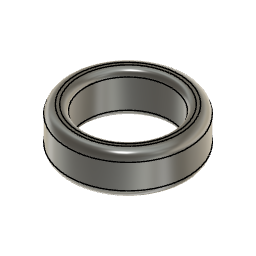
Anel_Redutor_Bracos_Imprimir (Autodesk Fusion 360 design; units mm, degrees)
Autodesk Fusion 360 part; units mm, degrees
sketch "Esboço1" plane through (0, 0, 0) normal (0, 0, 1) x (1, 0, 0)
  circle A0 centre (0, 0) radius 10.25
  circle A1 centre (0, 0) radius 14.5
  dimension "d1" = 20.5
  dimension "d2" = 4.25
  constraint coincident A0.centre A1.centre
  measures "d1" diameter of A0
extrude "Extrusão1" add sketch "Esboço1" along normal blind 10
fillet "Arredondamento1" radius 2 1 edges at (-13.5187, -5.2434, 10)
fillet "Arredondamento2" radius 2 1 edges at (-13.5187, -5.2434, 0)
fillet "Arredondamento3" radius 1.5 1 edges at (-9.5564, 3.7066, 10)
fillet "Arredondamento4" radius 1.5 1 edges at (-9.5564, 3.7066, 0)
